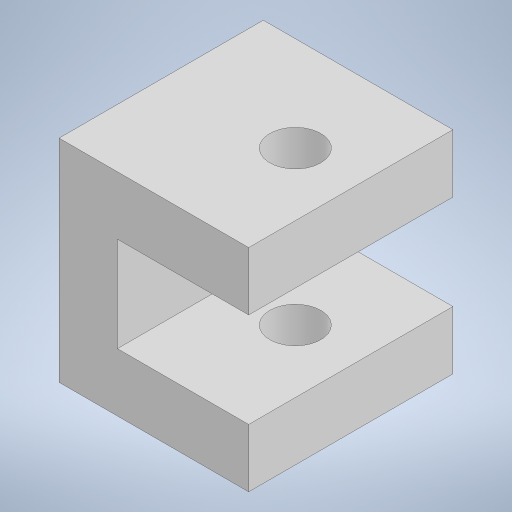
# Autodesk Inventor part: ограничитель
Saved by Autodesk Inventor 2023.1 (Build 271208000, 208)
## iProperties
Created: 2025-12-22
Part Number: ограничитель
Material: Типовые
Document SubType Name: Modeling
Designer: DELL
Density: 1 g/cm^3
Appearance: По умолчанию
Author: DELL
Autodesk Inventor part; units mm, degrees
ref_plane "YZ Plane" through (0, 0, 0) normal (1, 0, 0) x (0, 1, 0)
ref_plane "XZ Plane" through (0, 0, 0) normal (0, 1, 0) x (-1, 0, 0)
ref_plane "XY Plane" through (0, 0, 0) normal (0, 0, 1) x (1, 0, 0)
sketch "Эскиз2" plane through (0, 0, 0) normal (0, 0, 1) x (1, 0, 0)
  line L0 (-4.5, 3.25) -> (4.5, 3.25)
  line L1 (4.5, 3.25) -> (4.5, -3.25)
  line L2 (4.5, -3.25) -> (-4.5, -3.25)
  line L3 (-4.5, -3.25) -> (-4.5, 3.25)
  line L4 (-4.5, 3.25) -> (4.5, -3.25) construction
  line L5 (4.5, 3.25) -> (-4.5, -3.25) construction
  line L6 (8.5, 7.25) -> (4.5, 7.25) construction
  line L7 (-8.5, 7.25) -> (-8.5, -7.25)
  line L8 (-8.5, -7.25) -> (4.5, -7.25)
  line L9 (8.5, -7.25) -> (8.5, 7.25) construction
  line L10 (4.5, 3.25) -> (4.5, 7.25)
  line L11 (4.5, -3.25) -> (4.5, -7.25)
  line L12 (4.5, 7.25) -> (-8.5, 7.25)
  line L13 (4.5, -7.25) -> (8.5, -7.25) construction
  point P0 (0, 0)
  dimension "d0" = 9
  dimension "d1" = 6.5
  dimension "d2" = 4
  constraints: 28 end point, 7 parallel, 7 perpendicular, 2 midpoint, 1 horizontal
  measures "d0" distance of L1.end L2.end
  measures "d1" distance of L0.end L1.end
  measures "d2" distance between parallel lines of L0 L6
extrude "Выдавливание1" add sketch "Эскиз2" along normal blind 14 contours L3 L2 L11 L8 L7 L12 L10 L0
sketch "Эскиз3" plane through (-8.5, 7.25, 0) normal (0, 1, 0) x (1, 0, 0)
  line L0 (13, 0) -> (0, 0) construction
  circle A0 centre (8.695, -6.5) radius 1.75
  line L1 (13, 0) -> (13, -14) projected
  point P0 (8.5, 0)
  dimension "d5" = 3.5
  dimension "d9" = 4.305
  constraints: 1 centre point
  measures "d5" diameter of A0
  measures "d9" distance from line of L1 A0.centre
extrude "Выдавливание2" cut sketch "Эскиз3" against normal blind 20
